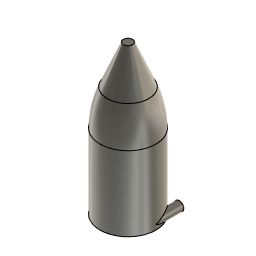
Vortex hangtime (Autodesk Fusion 360 design; units mm, degrees)
Autodesk Fusion 360 part; units mm, degrees
sketch "Sketch1" plane through (0, 0, 0) normal (0, 0, 1) x (1, 0, 0)
  circle A0 centre (0, 0) radius 60
  dimension "d1" = 120
  constraint coincident A0.centre origin
  measures "d1" diameter of A0
extrude "Extrude1" add sketch "Sketch1" along normal blind 200
sketch "Sketch2" plane through (0, 0, 0) normal (0, 1, 0) x (1, 0, 0)
  line L0 (70, -110) -> (70, -115.5379)
  line L1 (-60, -200) -> (-10, -320)
  line L2 (-10, -320) -> (0, -320)
  line L3 (0, -320) -> (0, -200)
  line L4 (0, -200) -> (-60, -200)
  constraint vertical L0
  constraint horizontal L2
  constraint perpendicular L2 L3
  constraint perpendicular L3 L4
revolve "Revolve1" add sketch "Sketch2" angle 360 about axis through (0, 0, 320) along (0, 0, -1)
fillet "Fillet1" radius 200 1 edges at (-55.9396, -21.6969, 200)
sketch "Sketch4" plane through (0, 0, 0) normal (0, 1, 0) x (1, 0, 0)
  circle A0 centre (50, -10) radius 10
extrude "Extrude2" add sketch "Sketch4" along normal blind 60
